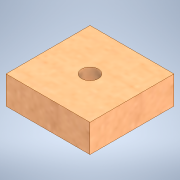
# Autodesk Inventor part: Box
Saved by Autodesk Inventor 2021 (Build 250183000, 183)
## iProperties
Created: 2021-07-05
Part Number: Box
Material: Wood (Cherry)
Document SubType Name: Modeling
Designer: KAVYA
Density: 0.63 g/cm^3
Appearance: Cherry - Natural Low Gloss
Author: KAVYA
Autodesk Inventor part; units mm, degrees
ref_plane "YZ Plane" through (0, 0, 0) normal (1, 0, 0) x (0, 1, 0)
ref_plane "XZ Plane" through (0, 0, 0) normal (0, 1, 0) x (-1, 0, 0)
ref_plane "XY Plane" through (0, 0, 0) normal (0, 0, 1) x (1, 0, 0)
sketch "Sketch1" plane through (0, 0, 0) normal (0, 1, 0) x (-1, 0, 0)
  line L0 (7.5385, 14.5615) -> (-22.4615, 14.5615)
  line L1 (-22.4615, 14.5615) -> (-22.4615, -15.4385)
  line L2 (-22.4615, -15.4385) -> (7.5385, -15.4385)
  line L3 (7.5385, -15.4385) -> (7.5385, 14.5615)
  point P0 (0, 0)
  dimension "d0" = 30
  dimension "d1" = 30
  constraints: 8 end point, 2 parallel, 1 horizontal, 1 perpendicular
  measures "d0" distance of L2.end L1.end
  measures "d1" distance of L1.end L0.end
extrude "Extrusion1" add sketch "Sketch1" along normal blind 10
sketch "Sketch2" plane through (0, 10, 0) normal (0, 1, 0) x (1, 0, 0)
  circle A0 centre (7.4615, 0.4385) radius 3
  line L0 (-7.5385, 15.4385) -> (-7.5385, -14.5615) projected
  line L1 (22.4615, 15.4385) -> (-7.5385, 15.4385) projected
  point P0 (0, 0)
  dimension "d4" = 6
  dimension "d5" = 15
  dimension "d6" = 15
  constraints: 1 centre point
  measures "d4" diameter of A0
  measures "d5" distance from line of A0.centre L0
  measures "d6" distance from line of L1 A0.centre
extrude "Extrusion2" cut sketch "Sketch2" against normal blind 5
body "Solid1"
